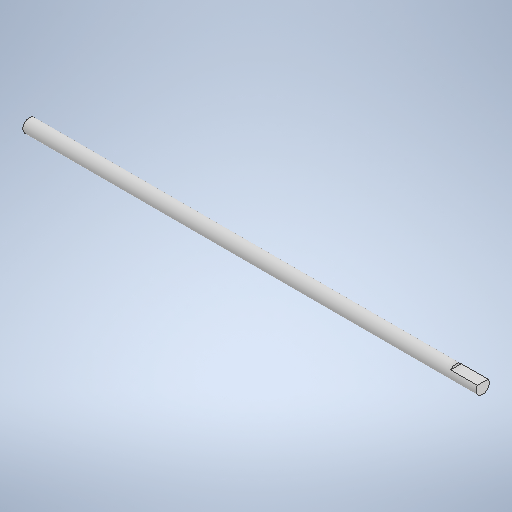
# Autodesk Inventor part: Eje 5mm
Saved by Autodesk Inventor 2025.3 (Build 293356000, 356)
## iProperties
Created: 2025-11-12
Part Number: Eje 5mm
Material: Generic
Document SubType Name: Modeling
Designer: juanm
Density: 1 g/cm^3
Appearance: Default
Author: juanm
Autodesk Inventor part; units mm, degrees
ref_plane "YZ Plane" through (0, 0, 0) normal (1, 0, 0) x (0, 1, 0)
ref_plane "XZ Plane" through (0, 0, 0) normal (0, 1, 0) x (-1, 0, 0)
ref_plane "XY Plane" through (0, 0, 0) normal (0, 0, 1) x (1, 0, 0)
sketch "Sketch1" plane through (0, 0, 0) normal (1, 0, 0) x (0, 1, 0)
  circle A0 centre (0, 0) radius 2.5
  dimension "d0" = 5
  constraints: 1 centre point, 1 coincident
  measures "d0" diameter of A0
extrude "Extrusion1" add sketch "Sketch1" along normal blind 170
sketch "Sketch2" plane through (170, 0, 0) normal (1, 0, 0) x (0, 0, -1)
  circle A0 centre (0, 0) radius 2.5 projected
  line L0 (-2, 1.5) -> (2, 1.5)
  dimension "d5" = 1.5
  constraints: 2 end point, 2 point on circle, 1 horizontal
  measures "d5" distance from line of point (0, 0) L0
extrude "Extrusion2" cut sketch "Sketch2" against normal blind 10 contours L0 A0 picked at (0.534, 1.6398)
body "Solid1"
